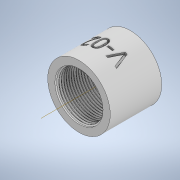
# Autodesk Inventor part: brakeStopAndOuterHousing
Saved by Autodesk Inventor 2021.1 (Build 251245000, 245)
## iProperties
Created: 2020-08-18
Part Number: brakeStopAndOuterHousing
Material: Generic
Document SubType Name: Modeling
Designer: robst
Density: 1 g/cm^3
Appearance: Default
Author: robst
Autodesk Inventor part; units mm, degrees
ref_plane "YZ Plane" through (0, 0, 0) normal (1, 0, 0) x (0, 1, 0)
ref_plane "XY Plane" through (0, 0, 0) normal (0, 0, 1) x (1, 0, 0)
sketch "Sketch3" plane through (0, 0, 0) normal (0, 0, 1) x (1, 0, 0)
  circle A0 centre (0, 0) radius 8.0645
  circle A1 centre (0, 0) radius 26.9875
  dimension "d8" = 16.129
  dimension "d9" = 53.975
  constraints: 2 centre point, 2 coincident
  measures "d8" diameter of A0
  measures "d9" diameter of A1
extrude "Extrusion3" add sketch "Sketch3" along normal blind 44.45
sketch "Sketch4" plane through (0, 0, 44.45) normal (0, 0, 1) x (1, 0, 0)
  circle A0 centre (0, 0) radius 20.7874
  dimension "d12" = 41.5747
  constraints: 1 centre point, 1 coincident
  measures "d12" diameter of A0
extrude "Extrusion4" cut sketch "Sketch4" against normal blind 31.75
sketch "Sketch5" plane through (0, 0, 0) normal (1, 0, 0) x (0, 1, 0)
  line L0 (20.7874, 44.45) -> (20.7874, 12.7) projected
  line L1 (26.9875, 44.45) -> (-26.9875, 44.45) projected
  line L2 (20.7874, 44.45) -> (20.7874, 44.45)
  line L3 (20.7874, 44.45) -> (19.6634, 43.8011)
  line L4 (19.6634, 43.6031) -> (20.7874, 42.9542)
  arc A0 (19.6634, 43.8011) -> (19.6634, 43.6031) centre (19.7206, 43.7021) ccw
  line L5 (0, -7.62) -> (0, 45.72) construction
  line L6 (20.7874, 42.9542) -> (20.7874, 44.45)
  point P0 (0, 0)
  dimension "d15" = 60
  dimension "d17" = 0.1143
  dimension "d18" = 19.6063
  dimension "d27" = 0
  constraints: 8 end point, 2 point on circle, 2 tangent, 1 centre point, 1 collinear, 1 equal length, 1 point on line, 1 vertical
  measures "d15" angle of L4 L3
  measures "d17" radius of A0
  measures "d18" distance edge to line of A0 L5
  measures "d27" distance of L2.end L0.start
coil "Coil2" sketch "Sketch5" operation add axis through (0, 0, -10) along (0, 0, -1) pitch 2.1167 turns 15 hand right
ref_plane "Work Plane1" through (0, 26.9875, 0) normal (0, 1, 0) x (-1, 0, 0)
ref_plane "Work Plane2" through (0, 26.9875, 0) normal (0, 1, 0) x (-1, 0, 0)
sketch "Sketch7" plane through (0, 26.9875, 0) normal (0, 1, 0) x (-1, 0, 0)
  line L0 (26.9875, 0) -> (26.9875, 44.45) projected
  line L1 (26.9875, 44.45) -> (-26.9875, 44.45) projected
  line L2 (-26.9875, 0) -> (-26.9875, 44.45) projected
  line L3 (-26.9875, 22.225) -> (26.9875, 22.225) construction
  line L4 (-7.4152, 28.575) -> (-11.7892, 15.875)
  line L5 (-11.7892, 15.875) -> (-13.6108, 15.875)
  line L6 (-13.6108, 15.875) -> (-17.9848, 28.575)
  line L7 (-17.9848, 28.575) -> (-16.1735, 28.575)
  line L8 (-16.1735, 28.575) -> (-12.6537, 18.026)
  line L9 (-12.6537, 18.026) -> (-9.1339, 28.575)
  line L10 (-9.1339, 28.575) -> (-7.4152, 28.575)
  line L11 (-1.765, 20.6607) -> (-6.5713, 20.6607)
  line L12 (-6.5713, 20.6607) -> (-6.5713, 22.2044)
  line L13 (-6.5713, 22.2044) -> (-1.765, 22.2044)
  line L14 (-1.765, 22.2044) -> (-1.765, 20.6607)
  spline S0 degree 2 poles (7.8269, 22.225) (7.8269, 18.8081) (5.8406, 15.6074) (3.7719, 15.6074) knots 0 0 0 1 2 2 2
  spline S1 degree 2 poles (3.7719, 15.6074) (1.6724, 15.6074) (-0.2933, 18.8699) (-0.2933, 22.2147) knots 0 0 0 1 2 2 2
  spline S2 degree 2 poles (-0.2933, 22.2147) (-0.2933, 25.6521) (1.693, 28.8323) (3.7719, 28.8323) knots 0 0 0 1 2 2 2
  spline S3 degree 2 poles (3.7719, 28.8323) (5.8611, 28.8323) (7.8269, 25.5389) (7.8269, 22.225) knots 0 0 0 1 2 2 2
  spline S4 degree 2 poles (5.645, 18.3553) (5.892, 18.9831) (6.0979, 20.9179) (6.0979, 22.225) knots 0 0 0 1 2 2 2
  spline S5 degree 2 poles (6.0979, 22.225) (6.0979, 23.5321) (5.892, 25.4566) (5.6347, 26.105) knots 0 0 0 1 2 2 2
  spline S6 degree 2 poles (5.6347, 26.105) (5.3774, 26.7534) (4.4821, 27.4223) (3.7719, 27.4223) knots 0 0 0 1 2 2 2
  spline S7 degree 2 poles (3.7719, 27.4223) (3.0618, 27.4223) (2.1458, 26.7534) (1.8782, 26.0844) knots 0 0 0 1 2 2 2
  spline S8 degree 2 poles (1.8782, 26.0844) (1.6209, 25.436) (1.4357, 23.46) (1.4357, 22.2147) knots 0 0 0 1 2 2 2
  spline S9 degree 2 poles (1.4357, 22.2147) (1.4357, 20.8768) (1.6004, 19.086) (1.868, 18.3862) knots 0 0 0 1 2 2 2
  spline S10 degree 2 poles (1.868, 18.3862) (2.115, 17.7275) (3.0309, 17.0174) (3.7719, 17.0174) knots 0 0 0 1 2 2 2
  spline S11 degree 2 poles (3.7719, 17.0174) (4.4718, 17.0174) (5.3877, 17.6863) (5.645, 18.3553) knots 0 0 0 1 2 2 2
  line L15 (17.285, 15.875) -> (9.453, 15.875)
  line L16 (9.453, 15.875) -> (9.453, 17.6761)
  spline S12 degree 2 poles (9.453, 17.6761) (10.2969, 18.4685) (11.7995, 19.9402) (12.5199, 20.7327) knots 0 0 0 1 2 2 2
  spline S13 degree 2 poles (12.5199, 20.7327) (13.971, 22.3279) (15.0311, 24.2422) (15.0311, 25.2611) knots 0 0 0 1 2 2 2
  spline S14 degree 2 poles (15.0311, 25.2611) (15.0311, 25.7962) (14.7017, 26.599) (14.4033, 26.8563) knots 0 0 0 1 2 2 2
  spline S15 degree 2 poles (14.4033, 26.8563) (14.1048, 27.1136) (13.3226, 27.3709) (12.8492, 27.3709) knots 0 0 0 1 2 2 2
  spline S16 degree 2 poles (12.8492, 27.3709) (12.3964, 27.3709) (11.4701, 27.1444) (11.0482, 26.9695) knots 0 0 0 1 2 2 2
  spline S17 degree 2 poles (11.0482, 26.9695) (10.688, 26.8254) (10.019, 26.4137) (9.8132, 26.2697) knots 0 0 0 1 2 2 2
  line L17 (9.8132, 26.2697) -> (9.7205, 26.2697)
  line L18 (9.7205, 26.2697) -> (9.7205, 28.081)
  spline S18 degree 2 poles (9.7205, 28.081) (10.2454, 28.3383) (12.1288, 28.8426) (12.9727, 28.8426) knots 0 0 0 1 2 2 2
  spline S19 degree 2 poles (12.9727, 28.8426) (14.7532, 28.8426) (16.7601, 26.9592) (16.7601, 25.3537) knots 0 0 0 1 2 2 2
  spline S20 degree 2 poles (16.7601, 25.3537) (16.7601, 24.6024) (16.4102, 23.3468) (16.1014, 22.8116) knots 0 0 0 1 2 2 2
  spline S21 degree 2 poles (16.1014, 22.8116) (15.7927, 22.2559) (14.8973, 21.165) (14.4033, 20.6401) knots 0 0 0 1 2 2 2
  spline S22 degree 2 poles (14.4033, 20.6401) (13.6005, 19.7653) (11.6348, 17.8922) (11.0482, 17.3467) knots 0 0 0 1 2 2 2
  line L19 (11.0482, 17.3467) -> (17.285, 17.3467)
  line L20 (17.285, 17.3467) -> (17.285, 15.875)
  point P0 (0, 0)
  constraints: 2 end point, 2 midpoint, 1 horizontal
emboss "Emboss1" sketch "Sketch7" operation cut depth 2.54 direction (0, -1, 0) wrap yes faces at (26.9, -2.1716, 29.6333)
equation "\"d8\" = innerDiameter"
equation "\"d9\" = outsideDiameter"
equation "\"d10\" = lengthOfBrakeStop"
equation "\"d12\" = b1MajorDiameterAvg"
equation "\"d13\" = depthOfThread"
equation "\"d17\" = b1RootRadiusAvg"
equation "\"d18\" = 0.5 * b1MinorDiameterAvg"
equation "\"d28\" = pitch"
equation "\"d29\" = depthOfThread"
equation "\"innerDiameter\" = 16.129"
equation "\"heightOfBrake\" = 6.35"
equation "\"majorDiameter\" = 41.22928"
equation "\"pitchDiameter\" = 39.85514"
equation "\"minorDiameter\" = 38.7096"
equation "\"crestFlat\" = 0.4318"
equation "\"rootRadius\" = 0.22352"
equation "\"threadDepth\" = 1.52146"
equation "\"outsideDiameter\" = 53.975"
equation "\"lengthOfBrakeStop\" = 44.45"
equation "\"depthOfThread\" = lengthOfBrakeStop - brakeStopLength"
equation "\"d36\" = 0.5 * outsideDiameter"
equation "\"brakeStopLength\" = 12.7"
equation "\"d48\" = 0.5 * outsideDiameter"
equation "\"b1MajorDiameterAvg\" = 41.57472"
equation "\"b1MinorDiameterAvg\" = 39.21252"
equation "\"b1RootRadiusAvg\" = 0.1143"
equation "\"pitch\" = 2.116667"
body "Solid2"
